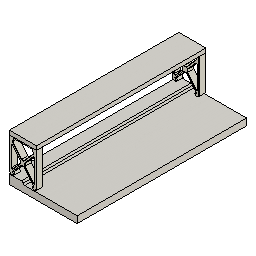
Planty Shelf v4 (Autodesk Fusion 360 design; units mm, degrees)
Autodesk Fusion 360 part; units mm, degrees
sketch "Sketch1" plane through (0, 0, 0) normal (0, 1, 0) x (1, 0, 0)
  line L0 (0, -7) -> (0, 0)
  line L1 (40, 0) -> (40, -7)
  line L2 (40, -7) -> (0, -7)
  line L3 (0, -119) -> (0, -107)
  line L4 (0, -107) -> (80, -107)
  line L5 (80, -107) -> (80, -119)
  line L6 (80, -119) -> (0, -119)
  line L7 (0, -107) -> (0, -7) construction
  line L8 (0, 0) -> (0, 20)
  line L9 (0, 20) -> (200, 20)
  line L10 (200, 20) -> (200, 0)
  line L11 (200, 0) -> (40, 0)
  line L12 (0, 0) -> (40, 0) construction
  dimension "d1" = 7
  dimension "d2" = 40
  dimension "d3" = 12
  dimension "d4" = 80
  dimension "d5" = 100
  dimension "d8" = 20
  dimension "d9" = 200
  constraint coincident L0.end L8.start
  constraint vertical L0
  constraint perpendicular L0 L2
  constraint vertical L3
  constraint perpendicular L3 L4
  constraint perpendicular L4 L5
  constraint horizontal L6
  constraint vertical L7
  constraint perpendicular L0 L9
  constraint perpendicular L1 L11
  constraint horizontal L11
  constraint vertical L10
  constraint horizontal L12
  constraint vertical L8
  measures "d1" distance of L1.start L1.end
  measures "d2" distance of L0.start L1.end
  measures "d3" distance of L3.start L3.end
  measures "d4" distance of L3.end L4.end
  measures "d5" distance of L0.start L3.end
  measures "d8" distance of L0.end L8.end
  measures "d9" distance of L8.end L9.end
extrude "Extrude1" add sketch "Sketch1" along normal blind 500 makes body 1 at (26.6667, 166.6667, 107) makes body 2 at (66.6667, 166.6667, -20) in component "Wood"
fillet "Fillet1" radius 5 1 edges at (40, 250, 7) on bodies 2 in component "Wood"
fillet "Fillet1" radius 5 1 edges at (40, 250, 0) on bodies 2 in component "Wood"
sketch "Sketch2" plane through (0, 0, 0) normal (0, 1, 0) x (1, 0, 0)
  line L0 (0, -107) -> (80, -107)
  line L1 (35.4606, -7) -> (0, -7)
  line L2 (200, 0) -> (45, 0)
  line L3 (0, -12) -> (35.4606, -12)
  line L4 (35.4606, -12) -> (45, -5)
  line L5 (45, -5) -> (80, -5)
  line L6 (80, -5) -> (80, -107)
  line L7 (0, -107) -> (0, -12)
  line L8 (35.4606, -12) -> (35.4606, -7) construction
  line L9 (45, -5) -> (45, 0) construction
  line L10 (0, -12) -> (5, -7)
  line L11 (15, -12) -> (10, -7)
  line L12 (80, -5) -> (75, 0)
  line L13 (70, 0) -> (65, -5)
  line L14 (5, -7) -> (10, -7)
  line L15 (70, 0) -> (75, 0)
  dimension "d14" = 5
  dimension "d15" = 5
  dimension "d16" = 45
  dimension "d17" = 45
  dimension "d18" = 5
  dimension "d19" = 45
  dimension "d20" = 45
  dimension "d21" = 5
  constraint horizontal L3
  constraint parallel L3 L5
  constraint coincident L0.end L6.end
  constraint perpendicular L3 L6
  constraint coincident L0.start L7.start
  constraint vertical L7
  constraint coincident L1.start L8.end
  constraint coincident L2.end L9.end
  constraint vertical L8
  constraint vertical L9
  constraint coincident L1 L10.end
  constraint coincident L3 L11.start
  constraint coincident L1 L11.end
  constraint coincident L2 L12.end
  constraint coincident L2 L13.start
  constraint coincident L5 L13.end
  measures "d14" distance of L1 L3
  measures "d15" distance of L2 L5
  measures "d16" angle of L3 L10
  measures "d17" angle of L3 L11
  measures "d18" distance of L10.end L11.end
  measures "d19" angle of L5 L13
  measures "d20" angle of L6 L12
  measures "d21" distance of L12.end L13.start
extrude "Extrude1'" add sketch "Sketch2" along normal blind 20 separate body makes body 3 in component "Shelf Leg"
sketch "Sketch3" plane through (0, 0, 0) normal (0, -1, 0) x (1, 0, 0)
  line L0 (10, 7) -> (15, 12)
  line L1 (15, 12) -> (35.4606, 12)
  line L2 (35.4606, 12) -> (45, 5)
  line L3 (45, 5) -> (65, 5)
  line L4 (65, 5) -> (70, 0)
  line L5 (70, 0) -> (75, 0)
  line L6 (75, 0) -> (80, 5)
  line L7 (80, 5) -> (80, 107)
  line L8 (80, 107) -> (0, 107)
  line L9 (0, 107) -> (0, 12)
  line L10 (0, 12) -> (5, 7)
  line L11 (5, 7) -> (10, 7)
  line L12 (6, 98) -> (74, 98)
  line L13 (74, 98) -> (74, 14)
  line L14 (6, 98) -> (6, 97.9533)
  line L15 (6, 97.9533) -> (6, 21)
  line L16 (65, 5) -> (74, 14)
  line L17 (15, 12) -> (6, 21)
  line L18 (6, 21) -> (74, 98)
  line L19 (10.2508, 16.7492) -> (74, 88.9358)
  line L20 (74, 14) -> (6, 98)
  line L21 (69.7339, 9.7339) -> (6, 88.4641)
  dimension "d24" = 6
  dimension "d25" = 6
  dimension "d26" = 9
  dimension "d29" = 6
  dimension "d30" = 6
  constraint horizontal L12
  constraint perpendicular L12 L13
  constraint perpendicular L12 L14
  constraint coincident L3.end L4.start
  constraint coincident L0.end L1.start
  constraint perpendicular L4 L16
  constraint perpendicular L0 L17
  constraint coincident L17 L19.start
  constraint parallel L18 L19
  constraint coincident L13 L19.end
  constraint coincident L16 L21.start
  constraint coincident L15 L21.end
  constraint parallel L20 L21
  measures "d24" distance of L9 L15
  measures "d25" distance of L7 L13
  measures "d26" distance of L8 L12
  measures "d29" distance of L18 L19
  measures "d30" distance of L20 L21
extrude "Extrude2" cut sketch "Sketch3" against normal through all contours L1 L2 L3 L16 L17 L19 L21 | L15 L18 L21 | L13 L19 L20 | L12 L18 L20 bodies 3 in component "Shelf Leg"
sketch "Sketch4" plane through (0, 0, 0) normal (-1, 0, 0) x (0, -1, 0)
  line L0 (0, 107) -> (0, 119)
  line L1 (0, 119) -> (-500, 119)
  line L2 (-500, 119) -> (-500, 107)
  line L3 (-500, 107) -> (0, 107)
  line L4 (-20, 98) -> (0, 98)
  line L5 (0, 98) -> (-20, 98)
  line L6 (-6.0397, 98.0603) -> (-0.1, 104)
  line L7 (-0.1, 104) -> (-6.0397, 104)
  line L8 (-6.0397, 104) -> (-6.0397, 98.0603)
  line L9 (-3.0698, 101.0302) -> (-16.5049, 114.4652)
  line L10 (0, 107) -> (-0.1, 104) construction
  dimension "d33" = 8.4
  dimension "d34" = 19
  dimension "d35" = 3
  dimension "d36" = 0.1
  constraint horizontal L7
  constraint perpendicular L7 L8
  constraint equal L7 L8
  constraint midpoint L6 L9.start
  constraint perpendicular L6 L9
  constraint coincident L0.start L3.end
  measures "d33" distance of L6.start L6.end
  measures "d34" distance of L9.start L9.end
  measures "d35" distance of L3 L7
  measures "d36" horizontal distance of L0.start L6.end
ref_plane "WorkPlane2" through (40, 0, 107) normal (0, 0.707107, 0.707107) x (1, 0, 0)
sketch "Sketch5" plane through (0, 0, 0) normal (1, 0, 0) x (0, 1, 0)
chamfer "Chamfer5" distance 5 angle 45 6 edges at (6, 10, 98) (74, 10, 98) (6, 10, 21) (74, 10, 14) (6, 10, 88.4641) (74, 10, 88.9358) tangent chain off on bodies 3 in component "Shelf Leg"
chamfer "Chamfer5" distance 5 angle 45 4 edges at (42.3501, 10, 53.0969) (38.5217, 10, 57.8261) (38.3225, 10, 48.5363) (34.4941, 10, 53.2654) tangent chain off on bodies 3 in component "Shelf Leg"
chamfer "Chamfer2" distance 6 angle 45 2 edges at (40, 0, 98) (40, 20, 98) on bodies 3 in component "Shelf Leg"
chamfer "Chamfer6" distance 1 angle 45 4 edges at (80, 20, 56) (0, 20, 59.5) (0, 0, 59.5) (80, 0, 56) on bodies 3 in component "Shelf Leg"
chamfer "Chamfer6" distance 2 angle 45 22 edges at (77.5, 20, 2.5) (72.5, 20, 0) (67.5, 20, 2.5) (67.367, 20, 7.367) (55.6012, 20, 27.192) (38.2406, 20, 44.7193) (22.6318, 20, 30.7688) (12.6254, 20, 14.3746) (12.5, 20, 9.5) (7.5, 20, 7) (2.5, 20, 9.5) (77.5, 0, 2.5) (72.5, 0, 0) (67.5, 0, 2.5) (67.367, 0, 7.367) (55.6012, 0, 27.192) (38.2406, 0, 44.7193) (22.6318, 0, 30.7688) (12.6254, 0, 14.3746) (12.5, 0, 9.5) (7.5, 0, 7) (2.5, 0, 9.5) on bodies 3 in component "Shelf Leg"
chamfer "Chamfer6" distance 1 angle 45 34 edges at (74, 20, 51.4679) (72.427, 20, 18.4431) (58.1751, 20, 33.5485) (45.578, 0, 53.0277) (45.578, 20, 53.0277) (58.1751, 20, 71.0164) (72.3451, 20, 84.5619) (58.1751, 0, 71.0164) (72.3451, 0, 84.5619) (74, 0, 51.4679) (72.427, 0, 18.4431) (58.1751, 0, 33.5485) (20.2471, 0, 70.8647) (31.2663, 0, 53.3346) (20.2471, 0, 37.1327) (7.6549, 0, 25.3739) (7.573, 0, 84.0209) (6, 0, 54.732) (56.2609, 0, 77.913) (22.2609, 0, 77.913) (38.6036, 0, 61.6431) (11.5042, 0, 99.0569) (68.4921, 0, 99.1261) (20.2471, 20, 70.8647) (7.573, 20, 84.0209) (6, 20, 54.732) (7.6549, 20, 25.3739) (20.2471, 20, 37.1327) (31.2663, 20, 53.3346) (38.6036, 20, 61.6431) (22.2609, 20, 77.913) (56.2609, 20, 77.913) (68.4921, 20, 99.1261) (11.5042, 20, 99.0569) on bodies 3 in component "Shelf Leg"
sketch "Sketch6" plane through (0, 52, 52) normal (0, -0.707107, -0.707107) x (1, 0, 0)
  line L0 (11, 65.0538) -> (69, 65.0538)
  line L1 (67.3909, 73.5391) -> (12.7545, 73.5391)
  line L2 (62, 69.2958) -> (18, 69.2958)
  line L3 (18, 65.0538) -> (18, 69.2958)
  line L4 (18, 69.2958) -> (0, 69.2958)
  line L5 (18, 69.2958) -> (18, 73.5391)
  line L6 (62, 69.2958) -> (80, 69.2958)
  line L7 (62, 69.2958) -> (62, 65.0538)
  line L8 (80, 3.5355) -> (80, 75.6604)
  line L9 (0, 75.6604) -> (0, 8.4853)
  line L10 (13.3854, 72.1249) -> (11, 65.0538)
  line L11 (69, 65.0538) -> (66.7449, 72.1249)
  line L12 (66.7449, 72.1249) -> (67.3909, 73.5391)
  line L13 (12.7545, 73.5391) -> (13.3854, 72.1249)
  dimension "d40" = 18
  dimension "d41" = 18
  dimension "d42" = 4.242
  dimension "d43" = 4.2433
  constraint parallel L0 L2
  constraint coincident L0 L3.start
  constraint perpendicular L2 L3
  constraint perpendicular L3 L4
  constraint coincident L1 L5.end
  constraint perpendicular L1 L5
  constraint parallel L2 L6
  constraint coincident L0 L7.end
  constraint perpendicular L0 L7
  constraint coincident L6.end L8
  constraint coincident L4.end L9
  measures "d40" distance of L2.start L6.end
  measures "d41" distance of L2.end L4.end
  measures "d42" distance of L2.end L3.start
  measures "d43" distance of L2.end L5.end
hole "Hole1" at (18, 3.0005, 100.9995) at (62, 3.0005, 100.9995) direction (0, 0.707107, 0.707107) diameter 4.5 depth 30 tip angle 180 countersink diameter 9.4 countersink angle 90 bodies 3 in component "Shelf Leg"
sketch "Sketch7" plane through (0, -42, 42) normal (0, 0.707107, -0.707107) x (-1, 0, 0)
  line L0 (-66.7449, 86.267) -> (-69, 79.196)
  line L1 (-69, 79.196) -> (-11, 79.196)
  line L2 (-11, 79.196) -> (-13.3854, 86.267)
  line L3 (-13.3854, 86.267) -> (-12.7545, 87.6812)
  line L4 (-12.7545, 87.6812) -> (-67.3909, 87.6812)
  line L5 (-67.3909, 87.6812) -> (-66.7449, 86.267)
  line L6 (-40.0727, 87.6812) -> (-40, 79.196)
  circle A0 centre (-40.0364, 83.4386) radius 2.1891
  constraint midpoint L4 L6.start
  constraint midpoint L1 L6.end
  constraint midpoint L6 A0.centre
hole "Hole2" at (40.0364, 17, 101) direction (0, -0.707107, 0.707107) diameter 4.5 depth 30 tip angle 180 countersink diameter 9.4 countersink angle 90 bodies 3 in component "Shelf Leg"
component "Wood" placed x (1, 0, 0) y (0, 1, 0) z (0, 0, 1) at (0, 0, 0)
component "Shelf Leg" placed x (1, 0, 0) y (0, 1, 0) z (0, 0, 1) at (0, 0, 0)
component "Shelf Leg" placed x (1, 0, 0) y (0, 1, 0) z (0, 0, 1) at (0, 480, 0)
equation "d16 = 45 °"
equation "d17 = 45 °"
equation "d19 = 45 °"
equation "d20 = 45.00 °"
